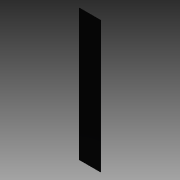
# Autodesk Inventor part: Feinte
Saved by Autodesk Inventor 2014 SP1 (Build 180222100, 222)
## iProperties
Created: 2015-03-28
Part Number: Feinte
Material: Generic
Document SubType Name: Modeling
Designer: tuleu
Density: 1 g/cm^3
Appearance: Default
Author: tuleu
Autodesk Inventor part; units mm, degrees
ref_plane "YZ Plane" through (0, 0, 0) normal (1, 0, 0) x (0, 1, 0)
ref_plane "XZ Plane" through (0, 0, 0) normal (0, 1, 0) x (-1, 0, 0)
ref_plane "XY Plane" through (0, 0, 0) normal (0, 0, 1) x (1, 0, 0)
sketch "Sketch1" plane through (0, 0, 0) normal (0, 1, 0) x (-1, 0, 0)
  line L0 (52.5, -322.5) -> (-52.5, -322.5)
  line L1 (-52.5, -322.5) -> (-52.5, 322.5)
  line L2 (-52.5, 322.5) -> (52.5, 322.5)
  line L3 (52.5, 322.5) -> (52.5, -322.5)
  line L4 (52.5, 0) -> (-52.5, 0)
  line L5 (0, -322.5) -> (0, 322.5)
  point P0 (0, 0)
  point P1 (0, 0)
  dimension "d0" = 105
  dimension "d1" = 645
  constraints: 12 end point, 5 midpoint, 3 perpendicular, 2 parallel, 1 coincident, 1 horizontal, 2 other
  measures "d0" distance of L0.start L0.end
  measures "d1" distance of L2.end L0.start
extrude "Extrusion1" add sketch "Sketch1" along normal blind 2
body "Solid1"
